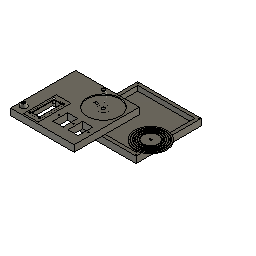
Untitled (Autodesk Fusion 360 design; units mm, degrees)
part number: 2025-10-25-14-32-45-415
Autodesk Fusion 360 part; units mm, degrees
note: some values were not read from the file. Chosen so that the rebuilt part matches the saved one: which bodies a step acts on; which face or edge a step refers to; which sketch regions a step uses. Set by a fixed rule: the direction of a hole.
sketch "Sketch1" plane through (0, 0, 0) normal (0, 0, 1) x (1, 0, 0)
sketch "Sketch2" plane through (0, 0, 0) normal (0, 0, 1) x (1, 0, 0)
  line L0 (-50, 50) -> (50, 50)
  line L1 (50, 50) -> (50, -50)
  line L2 (50, -50) -> (-50, -50)
  line L3 (-50, -50) -> (-50, 50)
  line L4 (-40, 40) -> (40, 40)
  line L5 (40, 40) -> (40, -40)
  line L6 (40, -40) -> (-40, -40)
  line L7 (-40, -40) -> (-40, 40)
  line L8 (-50, -50) -> (50, -50)
  line L9 (50, -50) -> (50, 50)
  line L10 (50, 50) -> (-50, 50)
  line L11 (-50, 50) -> (-50, -50)
  line L12 (50, -50) -> (0, -50)
  constraint horizontal L0
  constraint vertical L1
  constraint vertical L3
  constraint horizontal L4
  constraint vertical L5
  constraint horizontal L6
  constraint vertical L7
  constraint vertical L9
  constraint horizontal L10
  constraint vertical L11
sketch "Sketch3" plane through (0, 0, 10) normal (0, 0, 1) x (-1, 0, 0)
  line L0 (40, 40) -> (-40, 40)
  line L1 (-40, 40) -> (-40, -40)
  line L2 (-40, -40) -> (40, -40)
  line L3 (40, -40) -> (40, 40)
  line L4 (50, -50) -> (-50, -50)
  line L5 (-50, -50) -> (-50, 50)
  line L6 (-50, 50) -> (50, 50)
  line L7 (50, 50) -> (50, -50)
  constraint horizontal L4
  constraint vertical L5
  constraint horizontal L6
  constraint vertical L7
sketch "Sketch4" plane through (50, 0, 0) normal (1, 0, 0) x (0, 1, 0)
  line L0 (-50, 10) -> (50, 10)
  line L1 (50, 10) -> (50, 60)
  line L2 (50, 60) -> (-50, 60)
  line L3 (-50, 60) -> (-50, 10)
  circle A0 centre (0, 20) radius 5
  dimension "d5" = 10
  measures "d5" diameter of A0
sketch "Sketch8" plane through (0, 0, 0) normal (0, 0, 1) x (1, 0, 0)
  line L0 (-99.8621, 99.5976) -> (95.1379, 99.5976)
  line L1 (95.1379, 99.5976) -> (95.1379, -100.4024)
  line L2 (95.1379, -100.4024) -> (-99.8621, -100.4024)
  line L3 (-99.8621, -100.4024) -> (-99.8621, 99.5976)
  circle A0 centre (40.1379, 44.5976) radius 49.5
  circle A1 centre (47.5, -50) radius 42.5
  circle A2 centre (47.5, -50) radius 22.5
  circle A3 through (0.1806, 90, 0.1954) (-7.3194, 94.3301, 0.1954) (-7.3194, 85.6699, 0.1954)
  arc A4 through (36.1908, 50.2562, 8.3931) (20.1221, 75.3764, 7.5452) (-4.8194, 90, 0.1954)
  circle A5 centre (40.1379, 44.5976) radius 15
  line L4 (-65, 5) -> (-20, 5)
  line L5 (-20, 5) -> (-20, -95)
  line L6 (-20, -95) -> (-65, -95)
  line L7 (-65, -95) -> (-65, 5)
  line L8 (-50, 40) -> (-20, 40)
  line L9 (-20, 40) -> (-20, 15)
  line L10 (-20, 15) -> (-50, 15)
  line L11 (-50, 15) -> (-50, 40)
  circle A6 centre (-50, 27.5) radius 12.5
  circle A7 centre (-85, -75) radius 10
  circle A8 centre (-85, -75) radius 5
  dimension "d42" = 60
  dimension "d43" = 55
  dimension "d44" = 55
  dimension "d45" = 99
  dimension "d46" = 10
  dimension "d47" = 30
  constraint horizontal L0
  constraint vertical L1
  constraint horizontal L2
  constraint vertical L3
  constraint concentric A1 A2
  constraint concentric A0 A5
  constraint horizontal L4
  constraint vertical L5
  constraint horizontal L6
  constraint vertical L7
  constraint horizontal L8
  constraint vertical L9
  constraint horizontal L10
  constraint vertical L11
  constraint coincident L10.end A6
  constraint tangent L10 A6
  constraint coincident L8.start A6
  constraint concentric A7 A8
  measures "d42" distance of origin A0.centre
  measures "d43" distance of L1 A0.centre
  measures "d44" distance of L0 A0.centre
  measures "d45" diameter of A0
  measures "d47" diameter of A5
extrude "Extrude6" add sketch "Sketch8" against normal blind 50 contours L0 L1 L2 L3 makes body 1
extrude "Extrude7" add sketch "Sketch8" along normal blind -2 and the other way blind 50 contours A1 bodies 1
extrude "Extrude8" add sketch "Sketch8" against normal blind 40 contours A2 bodies 1
extrude "Extrude9" cut sketch "Sketch8" against normal blind 5 contours A2 bodies 1
extrude "Extrude10" add sketch "Sketch8" against normal blind 5 contours A2 bodies 1
extrude "Extrude11" cut sketch "Sketch8" against normal blind 1 contours A2 bodies 1
fillet "Fillet1" radius 1 2 edges at (26.5226, -58.1363, -2) (26.5226, -41.8637, -1) on bodies 1
extrude "Extrude12" add sketch "Sketch8" along normal blind -3 and the other way blind 50 contours A0 bodies 1
sketch "Sketch9" plane through (0, 0, 0.1954) normal (0, 0, 1) x (1, 0, 0)
sketch "Sketch8 (curves 0.1954 mm off its plane)" plane through (0, 0, 0.1954) normal (0, 0, 1) x (1, 0, 0)
  circle A0 centre (-4.8194, 90) radius 5
extrude "Extrude13" add sketch "Sketch8 (curves 0.1954 mm off its plane)" along normal blind -50 and the other way blind -2 bodies 1
extrude "Extrude14" add sketch "Sketch8" against normal blind 50 contours A5 bodies 1
pipe "Pipe1" add diameter 1.25 path "Sketch8" along A4 bodies 1
extrude "Extrude15" add sketch "Sketch8" along normal blind 5 and the other way blind 50 contours L4 L5 L6 L7 bodies 1
extrude "Extrude16" add sketch "Sketch8" against normal blind 50 contours A7 bodies 1
extrude "Extrude17" add sketch "Sketch8" against normal blind 50 contours A8 bodies 1
sketch "Sketch10" plane through (0, 0, 0) normal (0, 0, 1) x (1, 0, 0)
  circle A0 through (-80, -75, 9) (-87.5, -70.6699, 9) (-87.5, -79.3301, 9)
sketch "Sketch10 (curves 9 mm off its plane)" plane through (0, 0, 9) normal (0, 0, 1) x (1, 0, 0)
  circle A0 centre (-85, -75) radius 5
loft "Loft1" add profiles "Sketch8", "Sketch10 (curves 9 mm off its plane)" section 1 contours A7 section 2 bodies 1
extrude "Extrude18" add sketch "Sketch8" against normal blind 50 contours L11 A6 | L8 L9 L10 A6 | L11 A6 bodies 1
extrude "Extrude19" add sketch "Sketch8" along normal blind 3 contours L8 L9 L10 A6 bodies 1
extrude "Extrude20" add sketch "Sketch8" against normal blind 50 contours A2 bodies 1
sketch "Sketch11" plane through (0, 0, 0) normal (0, 0, 1) x (1, 0, 0)
  line L0 (-110, 110) -> (110, 110)
  line L1 (110, 110) -> (110, -110)
  line L2 (110, -110) -> (-110, -110)
  line L3 (-110, -110) -> (-110, 110)
  constraint horizontal L0
  constraint vertical L1
  constraint horizontal L2
  constraint vertical L3
move_body "Move1" bodies 1 to x (1, 0, 0) y (0, 1, 0) z (0, 0, 1) at (0, 0, -60)
extrude "Extrude21" add sketch "Sketch11" against normal blind 10 separate body makes body 2
move_body "Move2" bodies 1 to x (1, 0, 0) y (0, 1, 0) z (0, 0, 1) at (0, 0, 80)
combine "Combine1" operation cut target body 1 tool bodies 2 makes body 3 at (-34.8621, 32.931, -30)
hole "Hole1" at (91.7266, 96.0315, -30) direction (0, 0, 1) diameter 2.53 depth 30 tip angle 118 bodies 1 3
thread "Thread1" "ISO Metric profile 3.0 M3x0.5 M3x0.5 6H" thread offset 0 thread depth 7.4
hole "Hole2" at (91.9072, -97.0072, -30) direction (0, 0, 1) diameter 2.53 depth 25 tip angle 118 bodies 3
thread "Thread2" "ISO Metric profile 3.0 M3x0.5 M3x0.5 6H" thread offset 0 thread depth 7.4
hole "Hole3" at (-94.6479, 94.5231, -30) direction (0, 0, 1) diameter 2.53 depth 30 tip angle 118 bodies 1 3
thread "Thread3" "ISO Metric profile 3.0 M3x0.5 M3x0.5 6H" thread offset 0 thread depth 7.4
hole "Hole4" at (-94.624, -94.9374, -30) direction (0, 0, 1) diameter 2.53 depth 30 tip angle 118 bodies 1 3
thread "Thread4" "ISO Metric profile 3.0 M3x0.5 M3x0.5 6H" thread offset 0 thread depth 7.4
move_body "Move3" bodies 3 to x (1, 0, 0) y (0, 1, 0) z (0, 0, 1) at (180, 0, -100)
move_body "Move4" bodies 3 to x (1, 0, 0) y (0, 1, 0) z (0, 0, 1) at (15, -205, 0)
sketch "Sketch12" plane through (0, 0, -110) normal (0, 0, 1) x (-1, 0, 0)
  circle A0 centre (-100.376, 299.9374) radius 1.2645
  circle A1 centre (-100.3521, 110.4769) radius 1.2645
  circle A2 centre (-286.9072, 302.0072) radius 1.2645
  circle A3 centre (-286.7266, 108.9685) radius 1.2645
  line L0 (-290.1379, 305.4024) -> (-290.1379, 105.4024)
  line L1 (-290.1379, 105.4024) -> (-95.1379, 105.4024)
  line L2 (-95.1379, 105.4024) -> (-95.1379, 305.4024)
  line L3 (-95.1379, 305.4024) -> (-290.1379, 305.4024)
  line L4 (-280, 295) -> (-105, 295)
  line L5 (-105, 295) -> (-105, 115)
  line L6 (-105, 115) -> (-280, 115)
  line L7 (-280, 115) -> (-280, 295)
  constraint horizontal L4
  constraint vertical L5
  constraint horizontal L6
  constraint vertical L7
extrude "Extrude22" cut sketch "Sketch12" against normal blind 15 contours L4 L5 L6 L7 bodies 3
extrude "Extrude23" cut sketch "Sketch8" along normal blind 20 and the other way blind -17 contours A5 bodies 1
hole "Hole5" at (40.1379, 44.5976, 0) direction (0, 0, 1) diameter 10 depth 25 tip angle 180 bodies 1
extrude "Extrude24" cut sketch "Sketch8" along normal blind 15 contours A5 bodies 1
extrude "Extrude25" cut sketch "Sketch8" along normal blind 20 contours A1 | A2 bodies 1
sketch "Sketch13" plane through (0, 0, 20) normal (0, 0, 1) x (-1, 0, 0)
  arc A0 (50, -15) -> (50, -40) centre (50, -27.5) ccw
  line L0 (50, -40) -> (20, -40)
  line L1 (20, -40) -> (20, -15)
  line L2 (20, -15) -> (50, -15)
  circle A1 centre (85, 75) radius 10
  circle A2 centre (4.8194, -90) radius 5
  circle A3 centre (-40.1379, -44.5976) radius 49.5
  line L3 (20, 95) -> (65, 95)
  line L4 (65, 95) -> (65, -5)
  line L5 (65, -5) -> (20, -5)
  line L6 (20, -5) -> (20, 95)
  circle A4 centre (-47.5, 50) radius 42.5
  line L7 (99.8621, 100.4024) -> (-95.1379, 100.4024)
  line L8 (-95.1379, 100.4024) -> (-95.1379, -99.5976)
  line L9 (-95.1379, -99.5976) -> (99.8621, -99.5976)
  line L10 (99.8621, -99.5976) -> (99.8621, 100.4024)
  line L11 (-47.5, 50) -> (-47.5, 92.5)
  line L12 (-47.5, 50) -> (-90, 50)
  line L13 (-90, 92.5) -> (-47.5, 92.5)
  line L14 (-90, 92.5) -> (-90, 50)
  line L15 (-5, 92.5) -> (-5, 50)
  line L16 (-5, 92.5) -> (-47.5, 92.5)
  line L17 (-90, 7.5) -> (-90, 50)
  line L18 (-90, 7.5) -> (-47.5, 7.5)
  line L19 (-5, 7.5) -> (-47.5, 7.5)
  line L20 (-5, 7.5) -> (-5, 50)
  constraint coincident A4.centre L11.start
  constraint coincident A4 L11.end
  constraint vertical L11
  constraint coincident A4 L12.end
  constraint perpendicular L11 L12
  constraint tangent A4 L13
  constraint tangent A4 L14
  constraint symmetric L13.end L11 L16.end
  constraint symmetric L11 L12.end L15.end
  constraint symmetric L11 L13.start L15.start
  constraint symmetric L11.end L12 L18.end
  constraint symmetric L14.end L12 L17.end
  constraint symmetric L12 L13.start L17.start
  constraint symmetric L12 L15.start L19.start
  constraint symmetric L12 L15.end L20.end
  constraint symmetric L12 L11.end L18.end
hole "Hole6" at (90, -92.5, 20) direction (0, 0, -1) diameter 2.53 depth 3 tip angle 118 bodies 1
thread "Thread5" "ISO Metric profile 3.0 M3x0.5 M3x0.5 6H" thread offset 0 thread depth 7.4
hole "Hole7" at (90, -7.5, 20) direction (0, 0, -1) diameter 2.53 depth 3 tip angle 118 bodies 1
thread "Thread6" "ISO Metric profile 3.0 M3x0.5 M3x0.5 6H" thread offset 0 thread depth 7.4
hole "Hole8" at (5, -7.5, 20) direction (0, 0, -1) diameter 2.53 depth 3 tip angle 118 bodies 1
thread "Thread7" "ISO Metric profile 3.0 M3x0.5 M3x0.5 6H" thread offset 0 thread depth 7.4
hole "Hole9" at (5, -92.5, 20) direction (0, 0, -1) diameter 2.53 depth 3 tip angle 118 bodies 1
thread "Thread8" "ISO Metric profile 3.0 M3x0.5 M3x0.5 6H" thread offset 0 thread depth 7.4
extrude "Extrude26" cut 1 faces at (-50, -61.6667, 25) along direction (0, 0, -1) blind 30 on bodies 1 bodies 1
extrude "Extrude27" cut sketch "Sketch8" along normal blind 20 contours A7 | A8 bodies 1
extrude "Extrude28" cut sketch "Sketch8" along normal blind 22 contours A8 bodies 1
extrude "Extrude29" cut 1 faces at (-25.845, 27.8114, 23) along direction (0, 0, -1) blind 40 on bodies 1 bodies 1
extrude "Extrude30" cut sketch "Sketch8" along normal blind 19 contours L11 A6 picked at (-47.7473, 31.0052) bodies 1
sketch "Sketch14" plane through (0, 0, 17) normal (0, 0, 1) x (-1, 0, 0)
  circle A0 centre (-40.1379, -44.5976) radius 5
  circle A1 centre (-40.1379, -44.5976) radius 49.5
  line L0 (-20, -55) -> (-5, -55)
  line L1 (-5, -55) -> (-5, -45)
  line L2 (-5, -45) -> (-20, -45)
  line L3 (-20, -45) -> (-20, -55)
  constraint horizontal L0
  constraint vertical L1
  constraint horizontal L2
  constraint vertical L3
extrude "Extrude31" cut sketch "Sketch14" against normal blind 37 contours L0 L1 L2 L3 bodies 1
move_body "Move5" bodies 3 to x (1, 0, 0) y (0, 1, 0) z (0, 0, 1) at (60, 360, 0)
sketch "Sketch15" plane through (0, 0, 17) normal (0, 0, 1) x (-1, 0, 0)
  line L0 (-5, -55) -> (-20, -55)
  line L1 (-20, -55) -> (-20, -45)
  line L2 (-20, -45) -> (-5, -45)
  line L3 (-5, -45) -> (-5, -55)
  circle A0 centre (-40.1379, -44.5976) radius 5
  circle A1 centre (-40.1379, -44.5976) radius 49.5
  line L4 (-20, -45) -> (-10, -45)
  line L5 (-10, -45) -> (-10, -51)
  line L6 (-10, -51) -> (-20, -51)
  line L7 (-20, -51) -> (-20, -45)
  line L8 (-5, -55) -> (-20, -55)
  line L9 (-20, -55) -> (-20, -45)
  line L10 (-20, -45) -> (-5, -45)
  line L11 (-5, -45) -> (-5, -55)
  line L12 (-55, 50) -> (-24, 50)
  line L13 (-24, 50) -> (-24, 5)
  line L14 (-24, 5) -> (-55, 5)
  line L15 (-55, 5) -> (-55, 50)
  line L16 (-55, 50) -> (-86, 50)
  line L17 (-86, 50) -> (-86, 5)
  line L18 (-86, 5) -> (-55, 5)
  line L19 (-55, 5) -> (-55, 50)
  line L20 (-2.5826, 5) -> (-95, 5)
  line L21 (-95, 5) -> (-95, 100)
  line L22 (-95, 100) -> (-2.5826, 100)
  line L23 (-2.5826, 100) -> (-2.5826, 5)
  dimension "d159" = 10
  dimension "d160" = 31
  dimension "d161" = 45
  constraint horizontal L4
  constraint vertical L5
  constraint horizontal L6
  constraint vertical L7
  constraint coincident L1.end L2.start
  constraint horizontal L8
  constraint vertical L9
  constraint horizontal L10
  constraint vertical L11
  constraint coincident L0.start L3.end
  constraint horizontal L12
  constraint vertical L13
  constraint horizontal L14
  constraint vertical L15
  constraint horizontal L16
  constraint vertical L17
  constraint horizontal L18
  constraint vertical L19
  constraint horizontal L20
  constraint vertical L21
  constraint horizontal L22
  constraint vertical L23
  measures "d159" diameter of A0
  measures "d160" distance of L12.start L12.end
  measures "d161" distance of L12.start L14.end
extrude "Extrude32" add sketch "Sketch15" along normal blind -17 and the other way blind -3 contours L12 L13 L16 L17 L20 L21 L22 L23 bodies 1
extrude "Extrude33" add sketch "Sketch15" along normal blind -17 and the other way blind -3 contours L12 L13 L14 L15 L19 L20 | L15 L16 L17 L18 L19 L20 bodies 1
extrude "Extrude34" add sketch "Sketch15" against normal blind 17 separate body contours L0 L1 L2 L3 L5 L6 L8 L9 L10 L11 makes body 4
combine "Combine2" operation add target body 4 tool bodies 1
sketch "Sketch16" plane through (0, 0, 0) normal (0, 0, -1) x (1, 0, 0)
  line L0 (-50, -40) -> (-50, -15)
  line L1 (-50, -15) -> (-20, -15)
  line L2 (-20, -15) -> (-20, -40)
  line L3 (-20, -40) -> (-50, -40)
  circle A0 centre (-85, 75) radius 10
  line L4 (-20, 95) -> (-20, -5)
  line L5 (-20, -5) -> (-65, -5)
  line L6 (-65, -5) -> (-65, 95)
  line L7 (-65, 95) -> (-20, 95)
  circle A1 centre (40.1379, -44.5976) radius 15
  circle A2 centre (-94.624, 94.9374) radius 1.265
  circle A3 centre (-94.6479, -94.5231) radius 1.265
  circle A4 centre (91.7266, -96.0315) radius 1.265
  line L8 (95.1379, -99.5976) -> (95.1379, 100.4024)
  line L9 (95.1379, 100.4024) -> (-99.8621, 100.4024)
  line L10 (-99.8621, 100.4024) -> (-99.8621, -99.5976)
  line L11 (-99.8621, -99.5976) -> (95.1379, -99.5976)
  line L12 (10, -51) -> (10, -45)
  line L13 (10, -45) -> (20, -45)
  line L14 (20, -45) -> (20, -51)
  line L15 (20, -51) -> (10, -51)
  line L16 (7.5, -43) -> (22.5, -43)
  line L17 (22.5, -43) -> (22.5, -53)
  line L18 (22.5, -53) -> (7.5, -53)
  line L19 (7.5, -53) -> (7.5, -43)
  line L20 (20, -45) -> (10, -45)
  dimension "d172" = 15
  dimension "d173" = 10
  dimension "d174" = 2
  constraint horizontal L16
  constraint vertical L17
  constraint horizontal L18
  constraint vertical L19
  measures "d172" distance of L16.start L16.end
  measures "d173" distance of L16.start L18.end
  measures "d174" distance of L16 L20
extrude "Extrude35" cut sketch "Sketch16" against normal blind 4 contours L16 L17 L18 L19 bodies 4
sketch "Sketch17" plane through (0, 0, 20) normal (0, 0, 1) x (-1, 0, 0)
  line L0 (99.8621, 100.4024) -> (-95.1379, 100.4024)
  line L1 (-95.1379, 100.4024) -> (-95.1379, -99.5976)
  line L2 (-95.1379, -99.5976) -> (99.8621, -99.5976)
  line L3 (99.8621, -99.5976) -> (99.8621, 100.4024)
  line L4 (20, 95) -> (65, 95)
  line L5 (65, 95) -> (65, -5)
  line L6 (65, -5) -> (20, -5)
  line L7 (20, -5) -> (20, 95)
  circle A0 centre (-40.1379, -44.5976) radius 49.5
  circle A1 centre (4.8194, -90) radius 5
  circle A2 centre (85, 75) radius 10
  arc A3 (50, -15) -> (50, -40) centre (50, -27.5) ccw
  line L8 (50, -40) -> (20, -40)
  line L9 (20, -40) -> (20, -15)
  line L10 (20, -15) -> (50, -15)
  line L11 (0, 25) -> (-31, 25)
  line L12 (-31, 25) -> (-31, 70)
  line L13 (-31, 70) -> (0, 70)
  line L14 (0, 70) -> (0, 25)
  line L15 (-46, 25) -> (-77, 25)
  line L16 (-77, 25) -> (-77, 70)
  line L17 (-77, 70) -> (-46, 70)
  line L18 (-46, 70) -> (-46, 25)
  circle A4 centre (7.5, 45) radius 2.5
  line L19 (7.5, 47.5) -> (0, 52.5)
  line L20 (7.5, 42.5) -> (0, 37.5)
  line L21 (-38.5, 42.5) -> (-31, 37.5)
  circle A5 centre (-38.5, 45) radius 2.5
  line L22 (-38.5, 47.5) -> (-31, 52.5)
  line L23 (-38.5, 42.5) -> (-46, 37.5)
  line L24 (-38.5, 47.5) -> (-46, 52.5)
  circle A6 centre (-84.5, 45) radius 2.5
  line L25 (-84.5, 42.5) -> (-77, 37.5)
  line L26 (-84.5, 47.5) -> (-77, 52.5)
  dimension "d177" = 31
  dimension "d178" = 45
  dimension "d179" = 31
  dimension "d180" = 45
  dimension "d181" = 15
  dimension "d182" = 45
  dimension "d183" = 7.5
  dimension "d184" = 7.5
  dimension "d185" = 20
  constraint horizontal L11
  constraint vertical L12
  constraint horizontal L13
  constraint vertical L14
  constraint horizontal L15
  constraint vertical L16
  constraint horizontal L17
  constraint vertical L18
  constraint coincident A4 L19.start
  constraint coincident L14 L19.end
  constraint coincident A4 L20.start
  constraint coincident L14 L20.end
  constraint coincident L18 L23.end
  constraint coincident L18 L24.end
  measures "d177" distance of L11.start L11.end
  measures "d178" distance of L11.start L13.end
  measures "d179" distance of L15.start L15.end
  measures "d180" distance of L15.start L17.end
  measures "d181" distance of L12 L18
  measures "d182" distance of L15.end L16.end
  measures "d183" distance of L14 A4.centre
  measures "d184" horizontal distance of L19.start L19.end
  measures "d185" distance of L7 L14
hole "Hole10" at (-7.5, -45, 20) direction (0, 0, -1) diameter 3.78 depth 7 tip angle 118 bodies 4
thread "Thread9" "ISO Metric profile 4.5 M4.5x0.75 M4.5x0.75 6H" thread offset 0 thread depth 7.4
hole "Hole11" at (38.5, -45, 20) direction (0, 0, -1) diameter 3.78 depth 7 tip angle 118 bodies 4
thread "Thread10" "ISO Metric profile 4.5 M4.5x0.75 M4.5x0.75 6H" thread offset 0 thread depth 7.4
hole "Hole12" at (84.5, -45, 20) direction (0, 0, -1) diameter 3.78 depth 7 tip angle 118 bodies 4
thread "Thread11" "ISO Metric profile 4.5 M4.5x0.75 M4.5x0.75 6H" thread offset 0 thread depth 7.4
extrude "Extrude36" cut sketch "Sketch17" against normal blind 20 contours L11 L12 L13 L14 bodies 4
extrude "Extrude37" cut sketch "Sketch17" against normal blind 20 contours L15 L16 L17 L18 bodies 4
sketch "Sketch18" plane through (0, 0, 20) normal (0, 0, 1) x (-1, 0, 0)
  line L0 (20, -5) -> (65, -5)
  line L1 (65, -5) -> (65, 95)
  line L2 (65, 95) -> (20, 95)
  line L3 (20, 95) -> (20, -5)
  line L4 (26.5791, 5) -> (61.5791, 5)
  line L5 (61.5791, 5) -> (61.5791, 85)
  line L6 (61.5791, 85) -> (26.5791, 85)
  line L7 (26.5791, 85) -> (26.5791, 5)
  line L8 (20, 95) -> (65, 95)
  circle A0 centre (29.5791, 8) radius 3
  circle A1 centre (58.5791, 8) radius 3
  circle A2 centre (29.5791, 82) radius 3
  circle A3 centre (58.5791, 82) radius 3
  dimension "d206" = 35
  dimension "d207" = 80
  dimension "d208" = 10
  dimension "d209" = 10
  dimension "d210" = 10
  dimension "d211" = 3
  dimension "d214" = 29
  dimension "d215" = 74
  constraint horizontal L0
  constraint vertical L1
  constraint horizontal L2
  constraint vertical L3
  constraint horizontal L4
  constraint vertical L5
  constraint horizontal L6
  constraint vertical L7
  constraint tangent L4 A0
  constraint tangent L7 A0
  measures "d206" distance of L4.start L4.end
  measures "d207" distance of L4.start L6.end
  measures "d208" distance of L2 L6
  measures "d209" distance of L6 L8
  measures "d210" distance of L0 L4
  measures "d211" radius of A0
extrude "Extrude38" add sketch "Sketch18" against normal blind 20 separate body contours L0 L1 L2 L3 L8 | L4 L7 A0 | L4 L5 L6 L7 A0 A1 A2 A3 | A0 | L4 L5 A1 | A1 | L6 L7 A2 | A2 | L5 L6 A3 | A3 makes body 5
hole "Hole13" at (-29.5791, -8, 20) direction (0, 0, -1) diameter 6.04 depth 13 tip angle 118 bodies 5
thread "Thread12" "ISO Metric profile 7.0 M7x1 M7x1 6H" thread offset 0 thread depth 7.4
hole "Hole14" at (-58.5791, -8, 20) direction (0, 0, -1) diameter 6.04 depth 13 tip angle 118 bodies 5
thread "Thread13" "ISO Metric profile 7.0 M7x1 M7x1 6H" thread offset 0 thread depth 7.4
hole "Hole15" at (-29.5791, -82, 20) direction (0, 0, -1) diameter 6.04 depth 13 tip angle 118 bodies 5
thread "Thread14" "ISO Metric profile 7.0 M7x1 M7x1 6H" thread offset 0 thread depth 7.4
hole "Hole16" at (-58.5791, -82, 20) direction (0, 0, -1) diameter 6.04 depth 13 tip angle 118 bodies 5
thread "Thread15" "ISO Metric profile 7.0 M7x1 M7x1 6H" thread offset 0 thread depth 7.4
sketch "Sketch19" plane through (0, 0, 20) normal (0, 0, 1) x (-1, 0, 0)
  line L0 (32, 10) -> (56, 10)
  line L1 (56, 10) -> (56, 80)
  line L2 (56, 80) -> (32, 80)
  line L3 (32, 80) -> (32, 10)
  constraint horizontal L0
  constraint vertical L1
  constraint horizontal L2
  constraint vertical L3
extrude "Extrude39" add sketch "Sketch18" against normal blind 19 contours A0 | A1 | A2 | A3 bodies 5
extrude "Extrude40" cut sketch "Sketch19" against normal blind 83 bodies 5
extrude "Extrude41" cut sketch "Sketch18" along normal blind -2 and the other way blind 20 contours L4 L5 L6 L7 A0 A1 A2 A3 bodies 5
hole "Hole17" at (-29.5791, -8, 20) direction (0, 0, -1) diameter 5.04 depth 13 tip angle 118 bodies 5
thread "Thread16" "ISO Metric profile 6.0 M6x1 M6x1 6H" thread offset 0 thread depth 7.4
hole "Hole18" at (-58.5791, -8, 20) direction (0, 0, -1) diameter 5.04 depth 13 tip angle 118 bodies 5
thread "Thread17" "ISO Metric profile 6.0 M6x1 M6x1 6H" thread offset 0 thread depth 7.4
hole "Hole19" at (-29.5791, -82, 20) direction (0, 0, -1) diameter 5.04 depth 13 tip angle 118 bodies 5
thread "Thread18" "ISO Metric profile 6.0 M6x1 M6x1 6H" thread offset 0 thread depth 7.4
hole "Hole20" at (-58.5791, -82, 20) direction (0, 0, -1) diameter 5.04 depth 13 tip angle 118 bodies 5
thread "Thread19" "ISO Metric profile 6.0 M6x1 M6x1 6H" thread offset 0 thread depth 7.4
sketch "Sketch20" plane through (0, 0, 22) normal (0, 0, -1) x (1, 0, 0)
  circle A0 centre (-85, 75) radius 5
  circle A1 centre (-85, 75) radius 2.5
  circle A2 centre (-85, 75) radius 5
  constraint concentric A0 A1
  constraint concentric A1 A2
extrude "Extrude42" add sketch "Sketch20" along normal blind 2 separate body makes body 6
extrude "Extrude43" cut sketch "Sketch20" against normal blind 6.5 contours A1 bodies 4
sketch "Sketch21" plane through (0, 0, 20) normal (0, 0, -1) x (1, 0, 0)
  circle A0 centre (-85, 75) radius 2.5
  circle A1 centre (-85, 75) radius 5
  line L0 (-98.8924, 82.8964, 20) -> (-67.3625, 82.8964, 20)
  line L1 (-67.3625, 82.8964, 20) -> (-67.3625, 65.8964, 20)
  line L2 (-67.3625, 65.8964, 20) -> (-98.8924, 65.8964, 20)
  line L3 (-98.8924, 65.8964, 20) -> (-98.8924, 82.8964, 20)
  dimension "d270" = 17
sketch "Sketch21 (curves 20 mm off its plane)" plane through (0, 0, 0) normal (0, 0, -1) x (1, 0, 0)
  line L0 (-98.8924, 82.8964) -> (-67.3625, 82.8964)
  line L1 (-67.3625, 82.8964) -> (-67.3625, 65.8964)
  line L2 (-67.3625, 65.8964) -> (-98.8924, 65.8964)
  line L3 (-98.8924, 65.8964) -> (-98.8924, 82.8964)
extrude "Extrude44" cut sketch "Sketch21 (curves 20 mm off its plane)" against normal blind 14 bodies 4
extrude "Extrude45" add sketch "Sketch8" along normal blind 20 contours L11 A6 | L8 L9 L10 A6 picked at (-47.7473, 31.0052) bodies 4
sketch "Sketch22" plane through (0, 0, 20) normal (0, 0, 1) x (-1, 0, 0)
  circle A0 centre (85, 75) radius 10
  circle A1 centre (4.8194, -90) radius 5
  circle A2 centre (-40.1379, -44.5976) radius 49.5
  line L0 (20, 95) -> (65, 95)
  line L1 (65, 95) -> (65, -5)
  line L2 (65, -5) -> (20, -5)
  line L3 (20, -5) -> (20, 95)
  line L4 (99.8621, 100.4024) -> (-95.1379, 100.4024)
  line L5 (-95.1379, 100.4024) -> (-95.1379, -99.5976)
  line L6 (-95.1379, -99.5976) -> (99.8621, -99.5976)
  line L7 (99.8621, -99.5976) -> (99.8621, 100.4024)
  circle A3 centre (7.5, 45) radius 1.8915
  circle A4 centre (-38.5, 45) radius 1.8915
  circle A5 centre (-84.5, 45) radius 1.8915
  line L8 (-31, 25) -> (-31, 70)
  line L9 (-31, 70) -> (0, 70)
  line L10 (0, 70) -> (0, 25)
  line L11 (0, 25) -> (-31, 25)
  line L12 (-77, 25) -> (-77, 70)
  line L13 (-77, 70) -> (-46, 70)
  line L14 (-46, 70) -> (-46, 25)
  line L15 (-46, 25) -> (-77, 25)
  line L16 (20, -15) -> (62, -15)
  line L17 (62, -15) -> (62, -39)
  line L18 (62, -39) -> (20, -39)
  line L19 (20, -39) -> (20, -15)
  dimension "d275" = 42
  dimension "d276" = 24
  constraint horizontal L16
  constraint vertical L17
  constraint horizontal L18
  constraint vertical L19
  measures "d275" distance of L16.start L16.end
  measures "d276" distance of L16.start L18.end
move_body "Move6" bodies 3 to x (1, 0, 0) y (0, 1, 0) z (0, 0, 1) at (-260, 40, 0)
sketch "Sketch23" plane through (0, 0, 0) normal (0, 0, 1) x (1, 0, 0)
  line L0 (175, 50) -> (179.5, 50)
  line L1 (179.5, 50) -> (179.5, 46.2)
  line L2 (179.5, 46.2) -> (175, 46.2)
  line L3 (175, 46.2) -> (175, 50)
  circle A0 centre (179.5, 48.1) radius 1.9
  circle A1 centre (175, 48.1) radius 1.9
  dimension "d277" = 4.5
  dimension "d278" = 3.8
  constraint horizontal L0
  constraint vertical L1
  constraint horizontal L2
  constraint vertical L3
  constraint coincident L1.end A0
  constraint tangent L2 A0
  constraint coincident L0.end A0
  constraint coincident L2.end A1
  constraint tangent L2 A1
  constraint coincident L0.start A1
  measures "d277" distance of L0.start L0.end
  measures "d278" distance of L0.start L2.end
sketch "Sketch24" plane through (0, 0, 0) normal (0, 0, 1) x (1, 0, 0)
  circle A0 centre (177.25, 48.1) radius 49.25
  line L0 (179.5, 46.2) -> (175, 46.2)
  line L1 (175, 50) -> (179.5, 50)
  circle A1 centre (175, 48.1) radius 1.9
  circle A2 centre (179.5, 48.1) radius 1.9
  circle A3 centre (177.25, 48.1) radius 44.25
  circle A4 centre (177.25, 48.1) radius 39.25
  circle A5 centre (177.25, 48.1) radius 34.25
  circle A6 centre (177.25, 48.1) radius 29.25
  circle A7 centre (177.25, 48.1) radius 24.25
  dimension "d279" = 98.5
  dimension "d280" = 1.9
  dimension "d281" = 1.9
  dimension "d282" = 4.5
  dimension "d283" = 2.25
  dimension "d284" = 2.25
  dimension "d285" = 88.5
  dimension "d286" = 78.5
  dimension "d287" = 68.5
  dimension "d288" = 58.5
  dimension "d289" = 48.5
  constraint concentric A0 A3
  constraint concentric A3 A4
  constraint concentric A3 A5
  constraint concentric A3 A6
  constraint concentric A6 A7
  measures "d279" diameter of A0
  measures "d280" distance of A0.centre L0
  measures "d281" distance of A0.centre L1
  measures "d282" distance of A1.centre A2.centre
  measures "d283" distance of A0.centre A2.centre
  measures "d284" distance of A0.centre A1.centre
  measures "d285" diameter of A3
  measures "d286" diameter of A4
  measures "d287" diameter of A5
  measures "d288" diameter of A6
  measures "d289" diameter of A7
extrude "Extrude46" add sketch "Sketch23" sketch "Sketch24" along normal blind 3 separate body of sketch 2 contours A0 | L0 L1 A1 A2 | A2 | A1 | A3 | A4 | A5 | A6 | A7 makes body 7
extrude "Extrude47" cut sketch "Sketch24" along normal blind 10 contours L0 L1 A1 A2 | A2 | A1 bodies 7
pipe "Pipe2" cut diameter 1.5 path "Sketch24" along A7 bodies 7
pipe "Pipe3" cut diameter 1.5 path "Sketch24" along A6 bodies 7
pipe "Pipe4" cut diameter 1.5 path "Sketch24" along A5 bodies 7
pipe "Pipe5" cut diameter 1.5 path "Sketch24" along A4 bodies 7
pipe "Pipe6" cut diameter 1.5 path "Sketch24" along A3 bodies 7
move_body "Move7" bodies 7 to x (1, 0, 0) y (0, 1, 0) z (0, 0, 1) at (0, 0, -3)
pipe "Pipe7" cut diameter 1.5 path "Sketch24" along A7 bodies 7
pipe "Pipe8" cut diameter 1.5 path "Sketch24" along A6 bodies 7
pipe "Pipe9" cut diameter 1.5 path "Sketch24" along A5 bodies 7
pipe "Pipe10" cut diameter 1.5 path "Sketch24" along A4 bodies 7
pipe "Pipe11" cut diameter 1.5 path "Sketch24" along A3 bodies 7
sketch "Sketch25" plane through (0, 0, 0) normal (0, 0, 1) x (1, 0, 0)
  circle A0 centre (177.25, 48.1) radius 49.25
  line L0 (177.25, 48.1) -> (134.8112, 23.1097)
  line L1 (177.25, 48.1) -> (219.6888, 73.0902)
  dimension "d334" = 98.5
  constraint coincident A0.centre L0.start
  constraint coincident A0 L0.end
  constraint coincident A0 L1.end
  constraint parallel L0 L1
  measures "d334" diameter of A0
extrude "Extrude48" add sketch "Sketch25" against normal blind 1 contours A0 L0 L1 picked at (147.63, 62.0522) bodies 7
extrude "Extrude49" cut sketch "Sketch24" against normal blind 5 contours L0 L1 A1 A2 | A2 | A1 bodies 7
move_body "Move8" bodies 7 to x (-1, 0, 0) y (0, 1, 0) z (0, 0, -1) at (359, 0, 0)
